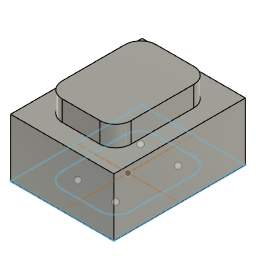
PCB Button (Autodesk Fusion 360 design; units mm, degrees)
Autodesk Fusion 360 part; units mm, degrees
sketch "Sketch1" plane through (0, 0, 0) normal (0, 0, 1) x (1, 0, 0)
  line L0 (41.7, -17.9) -> (45, -17.9)
  line L1 (45, -17.9) -> (45, -22.1)
  line L2 (45, -22.1) -> (41.7, -22.1)
  line L3 (41.7, -22.1) -> (41.7, -17.9)
  line L4 (42.75, -18.5) -> (43.95, -18.5)
  line L5 (44.45, -19) -> (44.45, -21)
  line L6 (43.95, -21.5) -> (42.75, -21.5)
  line L7 (42.25, -21) -> (42.25, -19)
  arc A0 (44.45, -19) -> (43.95, -18.5) centre (43.95, -19) ccw
  arc A1 (43.95, -21.5) -> (44.45, -21) centre (43.95, -21) ccw
  arc A2 (42.25, -21) -> (42.75, -21.5) centre (42.75, -21) ccw
  arc A3 (42.75, -18.5) -> (42.25, -19) centre (42.75, -19) ccw
  line L8 (43.35, -18.5) -> (43.35, -21.5) construction
  line L9 (42.25, -20) -> (44.45, -20) construction
  line L10 (41.7, -20) -> (45, -20) construction
  line L11 (43.35, -17.9) -> (43.35, -22.1) construction
  point P0 (43.35, -20)
  dimension "d365" = 4.2
  dimension "d366" = 3.3
  dimension "d367" = 3
  dimension "d368" = 2.2
  dimension "d369" = 0.5
  constraint horizontal L0
  constraint vertical L1
  constraint horizontal L2
  constraint vertical L3
  constraint horizontal L4
  constraint vertical L5
  constraint horizontal L6
  constraint vertical L7
  constraint tangent L4 A0
  constraint tangent L5 A0
  constraint tangent L5 A1
  constraint tangent L6 A1
  constraint equal A0 A1
  constraint tangent L6 A2
  constraint tangent L7 A2
  constraint equal A0 A2
  constraint tangent L4 A3
  constraint tangent L7 A3
  constraint equal A0 A3
  constraint midpoint L4 L8.start
  constraint midpoint L6 L8.end
  constraint midpoint L7 L9.start
  constraint midpoint L5 L9.end
  constraint midpoint L3 L10.start
  constraint midpoint L1 L10.end
  constraint midpoint L0 L11.start
  constraint midpoint L2 L11.end
  constraint midpoint L8 P0
  constraint coincident L10 P0
  constraint coincident L11 P0
  measures "d365" distance of L0 L2
  measures "d366" distance of L1 L3
  measures "d367" distance of L4 L6
  measures "d368" distance of L5 L7
  measures "d369" radius of A0
extrude "Extrude1" add sketch "Sketch1" along normal blind 1.85
extrude "Extrude2" add sketch "Sketch1" along normal blind 2.5 contours L4 L5 L6 L7 A0 A1 A2 A3
